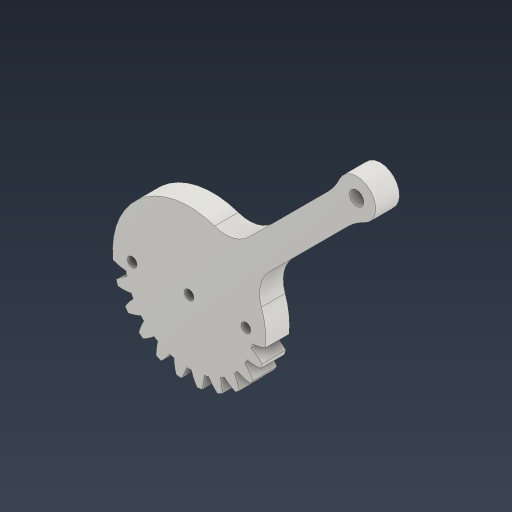
# Autodesk Inventor part: Zebatka_gut
Saved by Autodesk Inventor 2024 (Build 280153000, 153)
## iProperties
Created: 2023-12-19
Part Number: Zebatka_gut
Material: Steel
Document SubType Name: Modeling
Designer: Piter
Categories: <?xml version="1.0" encoding="UTF-16"?> <MemberInstance><Categories><FamilyTemplate><FamilyTemplateParameter ValueType="xs:double" Id="1" ObjectReferenceKey="da_z" ObjectType="kUserParameterObject"/><FamilyTemplateParameter ValueType="xs:double" Id="2" ObjectReferenceKey="da_b" ObjectType="kUserParameterObject"/><FamilyTemplateParameter ValueType="xs:double" Id="3" ObjectReferenceKey="da_beta" ObjectType="kUserParameterObject"/><FamilyTemplateParameter ValueType="xs:double" Id="4" ObjectReferenceKey="da_da" ObjectType="kUserParameterObject"/><FamilyTemplateParameter ValueType="xs:double" Id="5" ObjectReferenceKey="da_aw" ObjectType="kUserParameterObject"/><FamilyTemplateParameter ValueType="xs:string" Id="6" ObjectReferenceKey="EAIAABAAAACIAQAAAAAAAIAAAAAAAAAA" ObjectType="83910656" SubObjectId="SurfaceGeometry"/></FamilyTemplate><ParamToTemplateMap><ParamToTemplate CategoryParameter="//CategoryParameter[@InternalName='046C89C9-8512-4d59-83FE-43B91F4F132A']" TemplateParameter="1"/><ParamToTemplate CategoryParameter="//CategoryParameter[@InternalName='2552DF32-E462-4b46-AEBF-C6C7768E72AC']" TemplateParameter="2"/><ParamToTemplate CategoryParameter="//CategoryParameter[@InternalName='C9EE641D-15FC-4fae-A226-E94C4372FDD7']" TemplateParameter="3"/><ParamToTemplate><ParamToTemplate CategoryParameter="//CategoryParameter[@InternalName='00B6519A-459B-49c7-AD84-2E56D39A5744']" ConstantValue="0.571936"/></ParamToTemplate><ParamToTemplate><ParamToTemplate CategoryParameter="//CategoryParameter[@InternalName='04B31F0E-C7A6-4894-AA32-9629BEFACF47']" ConstantValue="1.000000"/></ParamToTemplate><ParamToTemplate><ParamToTemplate CategoryParameter="//CategoryParameter[@InternalName='43CBEC2E-7847-49e7-A936-2F7889FCB2D9']" ConstantValue="0.250000"/></ParamToTemplate><ParamToTemplate><ParamToTemplate CategoryParameter="//CategoryParameter[@InternalName='B1EFC894-105D-4ebd-86BF-FA20ED196853']" ConstantValue="0.350000"/></ParamToTemplate><ParamToTemplate><ParamToTemplate CategoryParameter="//CategoryParameter[@InternalName='51175063-3D10-4879-93E8-6246FE8B403D']" ConstantValue="2060000000.000000"/></ParamToTemplate><ParamToTemplate><ParamToTemplate CategoryParameter="//CategoryParameter[@InternalName='A3A52E27-4454-46a9-B0BD-C932399B70AF']" ConstantValue="0.300000"/></ParamToTemplate><ParamToTemplate><ParamToTemplate CategoryParameter="//CategoryParameter[@InternalName='91B76062-C214-41d9-B1B9-14D2AB99603D']" ConstantValue="0.125000"/></ParamToTemplate><ParamToTemplate><ParamToTemplate CategoryParameter="//CategoryParameter[@InternalName='374E806E-8B8A-4dda-A9AA-1039D6500AD2']" ConstantValue="8.000000"/></ParamToTemplate><ParamToTemplate><ParamToTemplate CategoryParameter="//CategoryParameter[@InternalName='2D373A89-B862-43d6-8D0B-0CBF12AB9F6C']" ConstantValue="0.349066"/></ParamToTemplate><ParamToTemplate CategoryParameter="//CategoryParameter[@InternalName='37777632-D6A2-4fac-9D53-DB8ACD95C989']" TemplateParameter="4"/><ParamToTemplate CategoryParameter="//CategoryParameter[@InternalName='FD1017F1-B727-4f7e-9707-0F86F1FF9423']" TemplateParameter="5"/><ParamToTemplate><ParamToTemplate CategoryParameter="//CategoryParameter[@InternalName='9E1B4470-B2D3-4ff1-B813-535BB4CDF51A']" ConstantValue="3520000.000000"/></ParamToTemplate><ParamToTemplate><ParamToTemplate CategoryParameter="//CategoryParameter[@InternalName='F8452263-BFF6-458c-9FB1-07C4B99E95CD']" ConstantValue="11400000.000000"/></ParamToTemplate><ParamToTemplate><ParamToTemplate CategoryParameter="//CategoryParameter[@InternalName='3E3BB259-FD49-497f-8171-6EBC954A3479']" ConstantValue="2.000000"/></ParamToTemplate><ParamToTemplate CategoryParameter="//CategoryParameter[@InternalName='27C3BAF2-7550-4e4b-AE2C-0DB134B7D9B7']" TemplateParameter="6"/></ParamToTemplateMap><Category DisplayName="Gear" InternalName="DC85795E-93AB-48d5-8EEE-5A27447B64BD" Mnemonic="Gear"><CategoryParameter DisplayName="z" InternalName="046C89C9-8512-4d59-83FE-43B91F4F132A" Mnemonic="z"/><CategoryParameter DisplayName="b" InternalName="2552DF32-E462-4b46-AEBF-C6C7768E72AC" Mnemonic="b"/><CategoryParameter DisplayName="||b|" InternalName="C9EE641D-15FC-4fae-A226-E94C4372FDD7" Mnemonic="beta"/><CategoryParameter DisplayName="x" InternalName="00B6519A-459B-49c7-AD84-2E56D39A5744" Mnemonic="x"/><CategoryParameter DisplayName="a*" InternalName="04B31F0E-C7A6-4894-AA32-9629BEFACF47" Mnemonic="a"/><CategoryParameter DisplayName="c*" InternalName="43CBEC2E-7847-49e7-A936-2F7889FCB2D9" Mnemonic="c"/><CategoryParameter DisplayName="r|.f|*" InternalName="B1EFC894-105D-4ebd-86BF-FA20ED196853" Mnemonic="rf"/><CategoryParameter DisplayName="E" InternalName="51175063-3D10-4879-93E8-6246FE8B403D" Mnemonic="E"/><CategoryParameter DisplayName="||m|" InternalName="A3A52E27-4454-46a9-B0BD-C932399B70AF" Mnemonic="mi"/><Category DisplayName="SpurGear" InternalName="26C5A22E-A91E-4dfd-A3B3-23CCAFAE1764" Mnemonic="SpurGear"><CategoryParameter DisplayName="m" InternalName="91B76062-C214-41d9-B1B9-14D2AB99603D" Mnemonic="m"/><CategoryParameter DisplayName="P" InternalName="374E806E-8B8A-4dda-A9AA-1039D6500AD2" Mnemonic="PP"/><CategoryParameter DisplayName="||a|" InternalName="2D373A89-B862-43d6-8D0B-0CBF12AB9F6C" Mnemonic="alpha"/><CategoryParameter DisplayName="d|.a|" InternalName="37777632-D6A2-4fac-9D53-DB8ACD95C989" Mnemonic="da"/><CategoryParameter DisplayName="a|.w|" InternalName="FD1017F1-B727-4f7e-9707-0F86F1FF9423" Mnemonic="aw"/><CategoryParameter DisplayName="||s||.Flim|" InternalName="9E1B4470-B2D3-4ff1-B813-535BB4CDF51A" Mnemonic="sFlim"/><CategoryParameter DisplayName="||s||.Hlim|" InternalName="F8452263-BFF6-458c-9FB1-07C4B99E95CD" Mnemonic="sHlim"/><CategoryParameter DisplayName="type" InternalName="3E3BB259-FD49-497f-8171-6EBC954A3479" Mnemonic="type"/><CategoryParameter DisplayName="PitchDiameter" InternalName="27C3BAF2-7550-4e4b-AE2C-0DB134B7D9B7" Mnemonic="IDS_PITCHDIAM"/></Category></Category></Categories></MemberInstance>
Density: 1 g/cm^3
Appearance: Steel
Author: Piter
Autodesk Inventor part; units mm, degrees
ref_plane "YZ Plane" through (0, 0, 0) normal (1, 0, 0) x (0, 1, 0)
ref_plane "XZ Plane" through (0, 0, 0) normal (0, 1, 0) x (-1, 0, 0)
ref_plane "XY Plane" through (0, 0, 0) normal (0, 0, 1) x (1, 0, 0)
sketch "Sketch1" plane through (0, 0, 0) normal (0, 0, 1) x (1, 0, 0)
  circle A0 centre (0, 0) radius 16.1601
  line L0 (0, 0) -> (14, 0)
  line L1 (14, 0) -> (-14, 0)
  line L2 (0, 0) -> (-12, 0)
  circle A1 centre (-12, 0) radius 1
  line L3 (0, 0) -> (0, 4.0083)
  circle A2 centre (12, 0) radius 1
  circle A3 centre (0, 0) radius 1
  dimension "d0" = 32.3202
  dimension "d53" = 12
  dimension "d54" = 2
  dimension "d57" = 2
  constraints: 8 end point, 4 centre point, 2 coincident, 2 point on line, 1 horizontal, 1 symmetric about line, 1 vertical, 1 other
  measures "d0" diameter of A0
  measures "d53" distance of L0.start L2.end
  measures "d54" diameter of A1
  measures "d57" diameter of A3
extrude "Extrusion1" add sketch "Sketch1" along normal blind 5
ref_plane "Work Plane2" through (0, 0, 2.5) normal (0, 0, 1) x (1, 0, 0)
sketch "Sketch2" plane through (0, 0, 0) normal (0, 0, -1) x (-1, 0, 0)
  circle A0 centre (0, 0) radius 16.1601 projected
  circle A1 centre (0, 0) radius 14.375
  dimension "d3" = 28.75
  constraints: 1 centre point, 1 coincident
  measures "d3" diameter of A1
surface extrude "Pitch Diameter" sketch "Sketch2" against normal through all shown no curves A1
ref_plane "Work Plane8" through (0, 0, 0) normal (0.9906859, 0.1361666, 0) x (0, 0, 1)
ref_plane "Work Plane9" through (0, 0, 0) normal (1, 0, 0) x (0, 1, 0)
spur gear teeth "Spur Gear" teeth 23 pitch diameter 28.75 tip diameter 32.3202 root diameter 27.0548 face width 20 start plane through (0, 0, 0) normal (0, 0, -1) x (-1, 0, 0)
sketch "Sketch3" plane through (0, 0, 5) normal (0, 0, 1) x (1, 0, 0)
  arc A0 (16.0754, -1.6526) -> (16.1507, -0.5517) centre (0, 0) ccw projected
  circle A1 centre (0, 0) radius 16.1601
  line L0 (-16.0754, -1.6526) -> (16.0754, -1.6526)
  arc A2 (16.1507, -0.5517) -> (13.5195, 0.4618) centre (11.2237, -9.4197) ccw projected
  circle A3 centre (0, 0) radius 13.5274
  line L1 (0, 0) -> (11.4269, -11.4269)
  line L2 (0, 0) -> (16.1601, 0) construction
  line L3 (9.1879, -4.9452) -> (4.9452, -9.1879)
  line L4 (9.1879, -4.9452) -> (4.9452, -9.1879)
  line L5 (4.9452, -9.1879) -> (33.234, -37.4767)
  line L6 (33.234, -37.4767) -> (37.4767, -33.234)
  line L7 (37.4767, -33.234) -> (9.1879, -4.9452)
  line L8 (0, 0) -> (28.7257, 0)
  line L9 (9.1879, 4.9452) -> (4.9452, 9.1879)
  line L10 (9.1879, 4.9452) -> (4.9452, 9.1879)
  line L11 (4.9452, 9.1879) -> (33.234, 37.4767)
  line L12 (33.234, 37.4767) -> (37.4767, 33.234)
  line L13 (37.4767, 33.234) -> (9.1879, 4.9452)
  circle A4 centre (35.3553, 35.3553) radius 4
  circle A5 centre (35.3553, 35.3553) radius 1.5
  point P0 (-13.4261, -1.6526)
  point P1 (11.2237, 9.4197)
  point P2 (11.4269, 11.4269)
  point P3 (9.107, 13.3496)
  point P4 (13.3496, 9.107)
  point P5 (35.6058, 31.3632)
  point P6 (31.3632, 35.6058)
  dimension "d58" = 45
  dimension "d59" = 3
  dimension "d60" = 3
  dimension "d62" = 8
  dimension "d63" = 3
  dimension "d65" = 50
  constraints: 28 end point, 6 symmetric about line, 4 equal length, 3 centre point, 3 coincident, 3 horizontal, 3 point on circle, 2 perpendicular, 1 midpoint, 3 other
  measures "d58" angle of L1 L2
  measures "d59" distance between parallel lines of L5 L1
  measures "d60" distance between parallel lines of L1 L7
  measures "d62" diameter of A4
  measures "d63" diameter of A5
  measures "d65" distance from line of L12 point (0, 0)
extrude "Extrusion2" add sketch "Sketch3" against normal blind 5 contours A2 L8 A1 | L8 A2 A3 L13 A1 | L13 A3 L11 A1 | A1 L11 A4 L13 | L0 A1 L11 A3 | A4 L11 L12 A5 L13 | L13 L12 A5 L11 A4
fillet "Fillet1" radius 7 2 edges at (9.107, 13.3496, 2.5) (13.3496, 9.107, 2.5)
fillet "Fillet2" radius 11.75 2 edges at (35.6058, 31.3632, 2.5) (31.3632, 35.6058, 2.5)
equation "\"d0\" = da_da"
equation "\"d3\" = da_d"
equation "\"da_da\" = 32.320161"
equation "\"da_d\" = 28.75"
body "Solid1"
body "Srf1"
